Autodesk Inventor part; units mm, degrees
(part 2 of 3)
ref_plane "to_Bolt_1_26_ZX" through (-239.759, 0, -300) normal (0, 0, -1) x (0, 1, 0)
ref_plane "to_Bolt_1_260_XY" through (-278.3133, 0, 300) normal (0, 1, 0) x (1, 0, 0)
ref_plane "to_Bolt_1_260_YZ" through (-278.3133, 0, 300) normal (1, 0, 0) x (0, 0, -1)
ref_plane "to_Bolt_1_260_ZX" through (-278.3133, 0, 300) normal (0, 0, -1) x (0, 1, 0)
ref_plane "to_Bolt_1_261_XY" through (-275.9036, 0, 300) normal (0, 1, 0) x (1, 0, 0)
ref_plane "to_Bolt_1_261_YZ" through (-275.9036, 0, 300) normal (1, 0, 0) x (0, 0, -1)
ref_plane "to_Bolt_1_261_ZX" through (-275.9036, 0, 300) normal (0, 0, -1) x (0, 1, 0)
ref_plane "to_Bolt_1_262_XY" through (-273.494, 0, 300) normal (0, 1, 0) x (1, 0, 0)
ref_plane "to_Bolt_1_262_YZ" through (-273.494, 0, 300) normal (1, 0, 0) x (0, 0, -1)
ref_plane "to_Bolt_1_262_ZX" through (-273.494, 0, 300) normal (0, 0, -1) x (0, 1, 0)
ref_plane "to_Bolt_1_263_XY" through (-271.0843, 0, 300) normal (0, 1, 0) x (1, 0, 0)
ref_plane "to_Bolt_1_263_YZ" through (-271.0843, 0, 300) normal (1, 0, 0) x (0, 0, -1)
ref_plane "to_Bolt_1_263_ZX" through (-271.0843, 0, 300) normal (0, 0, -1) x (0, 1, 0)
ref_plane "to_Bolt_1_264_XY" through (-268.6747, 0, 300) normal (0, 1, 0) x (1, 0, 0)
ref_plane "to_Bolt_1_264_YZ" through (-268.6747, 0, 300) normal (1, 0, 0) x (0, 0, -1)
ref_plane "to_Bolt_1_264_ZX" through (-268.6747, 0, 300) normal (0, 0, -1) x (0, 1, 0)
ref_plane "to_Bolt_1_265_XY" through (-266.2651, 0, 300) normal (0, 1, 0) x (1, 0, 0)
ref_plane "to_Bolt_1_265_YZ" through (-266.2651, 0, 300) normal (1, 0, 0) x (0, 0, -1)
ref_plane "to_Bolt_1_265_ZX" through (-266.2651, 0, 300) normal (0, 0, -1) x (0, 1, 0)
ref_plane "to_Bolt_1_266_XY" through (-263.8554, 0, 300) normal (0, 1, 0) x (1, 0, 0)
ref_plane "to_Bolt_1_266_YZ" through (-263.8554, 0, 300) normal (1, 0, 0) x (0, 0, -1)
ref_plane "to_Bolt_1_266_ZX" through (-263.8554, 0, 300) normal (0, 0, -1) x (0, 1, 0)
ref_plane "to_Bolt_1_267_XY" through (-261.4458, 0, 300) normal (0, 1, 0) x (1, 0, 0)
ref_plane "to_Bolt_1_267_YZ" through (-261.4458, 0, 300) normal (1, 0, 0) x (0, 0, -1)
ref_plane "to_Bolt_1_267_ZX" through (-261.4458, 0, 300) normal (0, 0, -1) x (0, 1, 0)
ref_plane "to_Bolt_1_268_XY" through (-259.0361, 0, 300) normal (0, 1, 0) x (1, 0, 0)
ref_plane "to_Bolt_1_268_YZ" through (-259.0361, 0, 300) normal (1, 0, 0) x (0, 0, -1)
ref_plane "to_Bolt_1_268_ZX" through (-259.0361, 0, 300) normal (0, 0, -1) x (0, 1, 0)
ref_plane "to_Bolt_1_269_XY" through (-256.6265, 0, 300) normal (0, 1, 0) x (1, 0, 0)
ref_plane "to_Bolt_1_269_YZ" through (-256.6265, 0, 300) normal (1, 0, 0) x (0, 0, -1)
ref_plane "to_Bolt_1_269_ZX" through (-256.6265, 0, 300) normal (0, 0, -1) x (0, 1, 0)
ref_plane "to_Bolt_1_27_XY" through (-237.3494, 0, -300) normal (0, 1, 0) x (1, 0, 0)
ref_plane "to_Bolt_1_27_YZ" through (-237.3494, 0, -300) normal (1, 0, 0) x (0, 0, -1)
ref_plane "to_Bolt_1_27_ZX" through (-237.3494, 0, -300) normal (0, 0, -1) x (0, 1, 0)
ref_plane "to_Bolt_1_270_XY" through (-254.2169, 0, 300) normal (0, 1, 0) x (1, 0, 0)
ref_plane "to_Bolt_1_270_YZ" through (-254.2169, 0, 300) normal (1, 0, 0) x (0, 0, -1)
ref_plane "to_Bolt_1_270_ZX" through (-254.2169, 0, 300) normal (0, 0, -1) x (0, 1, 0)
ref_plane "to_Bolt_1_271_XY" through (-251.8072, 0, 300) normal (0, 1, 0) x (1, 0, 0)
ref_plane "to_Bolt_1_271_YZ" through (-251.8072, 0, 300) normal (1, 0, 0) x (0, 0, -1)
ref_plane "to_Bolt_1_271_ZX" through (-251.8072, 0, 300) normal (0, 0, -1) x (0, 1, 0)
ref_plane "to_Bolt_1_272_XY" through (-249.3976, 0, 300) normal (0, 1, 0) x (1, 0, 0)
ref_plane "to_Bolt_1_272_YZ" through (-249.3976, 0, 300) normal (1, 0, 0) x (0, 0, -1)
ref_plane "to_Bolt_1_272_ZX" through (-249.3976, 0, 300) normal (0, 0, -1) x (0, 1, 0)
ref_plane "to_Bolt_1_273_XY" through (-246.988, 0, 300) normal (0, 1, 0) x (1, 0, 0)
ref_plane "to_Bolt_1_273_YZ" through (-246.988, 0, 300) normal (1, 0, 0) x (0, 0, -1)
ref_plane "to_Bolt_1_273_ZX" through (-246.988, 0, 300) normal (0, 0, -1) x (0, 1, 0)
ref_plane "to_Bolt_1_274_XY" through (-244.5783, 0, 300) normal (0, 1, 0) x (1, 0, 0)
ref_plane "to_Bolt_1_274_YZ" through (-244.5783, 0, 300) normal (1, 0, 0) x (0, 0, -1)
ref_plane "to_Bolt_1_274_ZX" through (-244.5783, 0, 300) normal (0, 0, -1) x (0, 1, 0)
ref_plane "to_Bolt_1_275_XY" through (-242.1687, 0, 300) normal (0, 1, 0) x (1, 0, 0)
ref_plane "to_Bolt_1_275_YZ" through (-242.1687, 0, 300) normal (1, 0, 0) x (0, 0, -1)
ref_plane "to_Bolt_1_275_ZX" through (-242.1687, 0, 300) normal (0, 0, -1) x (0, 1, 0)
ref_plane "to_Bolt_1_276_XY" through (-239.759, 0, 300) normal (0, 1, 0) x (1, 0, 0)
ref_plane "to_Bolt_1_276_YZ" through (-239.759, 0, 300) normal (1, 0, 0) x (0, 0, -1)
ref_plane "to_Bolt_1_276_ZX" through (-239.759, 0, 300) normal (0, 0, -1) x (0, 1, 0)
ref_plane "to_Bolt_1_277_XY" through (-237.3494, 0, 300) normal (0, 1, 0) x (1, 0, 0)
ref_plane "to_Bolt_1_277_YZ" through (-237.3494, 0, 300) normal (1, 0, 0) x (0, 0, -1)
ref_plane "to_Bolt_1_277_ZX" through (-237.3494, 0, 300) normal (0, 0, -1) x (0, 1, 0)
ref_plane "to_Bolt_1_278_XY" through (-234.9398, 0, 300) normal (0, 1, 0) x (1, 0, 0)
ref_plane "to_Bolt_1_278_YZ" through (-234.9398, 0, 300) normal (1, 0, 0) x (0, 0, -1)
ref_plane "to_Bolt_1_278_ZX" through (-234.9398, 0, 300) normal (0, 0, -1) x (0, 1, 0)
ref_plane "to_Bolt_1_279_XY" through (-232.5301, 0, 300) normal (0, 1, 0) x (1, 0, 0)
ref_plane "to_Bolt_1_279_YZ" through (-232.5301, 0, 300) normal (1, 0, 0) x (0, 0, -1)
ref_plane "to_Bolt_1_279_ZX" through (-232.5301, 0, 300) normal (0, 0, -1) x (0, 1, 0)
ref_plane "to_Bolt_1_28_XY" through (-234.9398, 0, -300) normal (0, 1, 0) x (1, 0, 0)
ref_plane "to_Bolt_1_28_YZ" through (-234.9398, 0, -300) normal (1, 0, 0) x (0, 0, -1)
ref_plane "to_Bolt_1_28_ZX" through (-234.9398, 0, -300) normal (0, 0, -1) x (0, 1, 0)
ref_plane "to_Bolt_1_280_XY" through (-230.1205, 0, 300) normal (0, 1, 0) x (1, 0, 0)
ref_plane "to_Bolt_1_280_YZ" through (-230.1205, 0, 300) normal (1, 0, 0) x (0, 0, -1)
ref_plane "to_Bolt_1_280_ZX" through (-230.1205, 0, 300) normal (0, 0, -1) x (0, 1, 0)
ref_plane "to_Bolt_1_281_XY" through (-227.7108, 0, 300) normal (0, 1, 0) x (1, 0, 0)
ref_plane "to_Bolt_1_281_YZ" through (-227.7108, 0, 300) normal (1, 0, 0) x (0, 0, -1)
ref_plane "to_Bolt_1_281_ZX" through (-227.7108, 0, 300) normal (0, 0, -1) x (0, 1, 0)
ref_plane "to_Bolt_1_282_XY" through (-225.3012, 0, 300) normal (0, 1, 0) x (1, 0, 0)
ref_plane "to_Bolt_1_282_YZ" through (-225.3012, 0, 300) normal (1, 0, 0) x (0, 0, -1)
ref_plane "to_Bolt_1_282_ZX" through (-225.3012, 0, 300) normal (0, 0, -1) x (0, 1, 0)
ref_plane "to_Bolt_1_283_XY" through (-222.8916, 0, 300) normal (0, 1, 0) x (1, 0, 0)
ref_plane "to_Bolt_1_283_YZ" through (-222.8916, 0, 300) normal (1, 0, 0) x (0, 0, -1)
ref_plane "to_Bolt_1_283_ZX" through (-222.8916, 0, 300) normal (0, 0, -1) x (0, 1, 0)
ref_plane "to_Bolt_1_284_XY" through (-220.4819, 0, 300) normal (0, 1, 0) x (1, 0, 0)
ref_plane "to_Bolt_1_284_YZ" through (-220.4819, 0, 300) normal (1, 0, 0) x (0, 0, -1)
ref_plane "to_Bolt_1_284_ZX" through (-220.4819, 0, 300) normal (0, 0, -1) x (0, 1, 0)
ref_plane "to_Bolt_1_285_XY" through (-218.0723, 0, 300) normal (0, 1, 0) x (1, 0, 0)
ref_plane "to_Bolt_1_285_YZ" through (-218.0723, 0, 300) normal (1, 0, 0) x (0, 0, -1)
ref_plane "to_Bolt_1_285_ZX" through (-218.0723, 0, 300) normal (0, 0, -1) x (0, 1, 0)
ref_plane "to_Bolt_1_286_XY" through (-215.6627, 0, 300) normal (0, 1, 0) x (1, 0, 0)
ref_plane "to_Bolt_1_286_YZ" through (-215.6627, 0, 300) normal (1, 0, 0) x (0, 0, -1)
ref_plane "to_Bolt_1_286_ZX" through (-215.6627, 0, 300) normal (0, 0, -1) x (0, 1, 0)
ref_plane "to_Bolt_1_287_XY" through (-213.253, 0, 300) normal (0, 1, 0) x (1, 0, 0)
ref_plane "to_Bolt_1_287_YZ" through (-213.253, 0, 300) normal (1, 0, 0) x (0, 0, -1)
ref_plane "to_Bolt_1_287_ZX" through (-213.253, 0, 300) normal (0, 0, -1) x (0, 1, 0)
ref_plane "to_Bolt_1_288_XY" through (-210.8434, 0, 300) normal (0, 1, 0) x (1, 0, 0)
ref_plane "to_Bolt_1_288_YZ" through (-210.8434, 0, 300) normal (1, 0, 0) x (0, 0, -1)
ref_plane "to_Bolt_1_288_ZX" through (-210.8434, 0, 300) normal (0, 0, -1) x (0, 1, 0)
ref_plane "to_Bolt_1_289_XY" through (-208.4337, 0, 300) normal (0, 1, 0) x (1, 0, 0)
ref_plane "to_Bolt_1_289_YZ" through (-208.4337, 0, 300) normal (1, 0, 0) x (0, 0, -1)
ref_plane "to_Bolt_1_289_ZX" through (-208.4337, 0, 300) normal (0, 0, -1) x (0, 1, 0)
ref_plane "to_Bolt_1_29_XY" through (-232.5301, 0, -300) normal (0, 1, 0) x (1, 0, 0)
ref_plane "to_Bolt_1_29_YZ" through (-232.5301, 0, -300) normal (1, 0, 0) x (0, 0, -1)
ref_plane "to_Bolt_1_29_ZX" through (-232.5301, 0, -300) normal (0, 0, -1) x (0, 1, 0)
ref_plane "to_Bolt_1_290_XY" through (-206.0241, 0, 300) normal (0, 1, 0) x (1, 0, 0)
ref_plane "to_Bolt_1_290_YZ" through (-206.0241, 0, 300) normal (1, 0, 0) x (0, 0, -1)
ref_plane "to_Bolt_1_290_ZX" through (-206.0241, 0, 300) normal (0, 0, -1) x (0, 1, 0)
ref_plane "to_Bolt_1_291_XY" through (-203.6145, 0, 300) normal (0, 1, 0) x (1, 0, 0)
ref_plane "to_Bolt_1_291_YZ" through (-203.6145, 0, 300) normal (1, 0, 0) x (0, 0, -1)
ref_plane "to_Bolt_1_291_ZX" through (-203.6145, 0, 300) normal (0, 0, -1) x (0, 1, 0)
ref_plane "to_Bolt_1_292_XY" through (-201.2048, 0, 300) normal (0, 1, 0) x (1, 0, 0)
ref_plane "to_Bolt_1_292_YZ" through (-201.2048, 0, 300) normal (1, 0, 0) x (0, 0, -1)
ref_plane "to_Bolt_1_292_ZX" through (-201.2048, 0, 300) normal (0, 0, -1) x (0, 1, 0)
ref_plane "to_Bolt_1_293_XY" through (-198.7952, 0, 300) normal (0, 1, 0) x (1, 0, 0)
ref_plane "to_Bolt_1_293_YZ" through (-198.7952, 0, 300) normal (1, 0, 0) x (0, 0, -1)
ref_plane "to_Bolt_1_293_ZX" through (-198.7952, 0, 300) normal (0, 0, -1) x (0, 1, 0)
ref_plane "to_Bolt_1_294_XY" through (-196.3855, 0, 300) normal (0, 1, 0) x (1, 0, 0)
ref_plane "to_Bolt_1_294_YZ" through (-196.3855, 0, 300) normal (1, 0, 0) x (0, 0, -1)
ref_plane "to_Bolt_1_294_ZX" through (-196.3855, 0, 300) normal (0, 0, -1) x (0, 1, 0)
ref_plane "to_Bolt_1_295_XY" through (-193.9759, 0, 300) normal (0, 1, 0) x (1, 0, 0)
ref_plane "to_Bolt_1_295_YZ" through (-193.9759, 0, 300) normal (1, 0, 0) x (0, 0, -1)
ref_plane "to_Bolt_1_295_ZX" through (-193.9759, 0, 300) normal (0, 0, -1) x (0, 1, 0)
ref_plane "to_Bolt_1_296_XY" through (-191.5663, 0, 300) normal (0, 1, 0) x (1, 0, 0)
ref_plane "to_Bolt_1_296_YZ" through (-191.5663, 0, 300) normal (1, 0, 0) x (0, 0, -1)
ref_plane "to_Bolt_1_296_ZX" through (-191.5663, 0, 300) normal (0, 0, -1) x (0, 1, 0)
ref_plane "to_Bolt_1_297_XY" through (-189.1566, 0, 300) normal (0, 1, 0) x (1, 0, 0)
ref_plane "to_Bolt_1_297_YZ" through (-189.1566, 0, 300) normal (1, 0, 0) x (0, 0, -1)
ref_plane "to_Bolt_1_297_ZX" through (-189.1566, 0, 300) normal (0, 0, -1) x (0, 1, 0)
ref_plane "to_Bolt_1_298_XY" through (-186.747, 0, 300) normal (0, 1, 0) x (1, 0, 0)
ref_plane "to_Bolt_1_298_YZ" through (-186.747, 0, 300) normal (1, 0, 0) x (0, 0, -1)
ref_plane "to_Bolt_1_298_ZX" through (-186.747, 0, 300) normal (0, 0, -1) x (0, 1, 0)
ref_plane "to_Bolt_1_299_XY" through (-184.3373, 0, 300) normal (0, 1, 0) x (1, 0, 0)
ref_plane "to_Bolt_1_299_YZ" through (-184.3373, 0, 300) normal (1, 0, 0) x (0, 0, -1)
ref_plane "to_Bolt_1_299_ZX" through (-184.3373, 0, 300) normal (0, 0, -1) x (0, 1, 0)
ref_plane "to_Bolt_1_3_XY" through (-295.1807, 0, -300) normal (0, 1, 0) x (1, 0, 0)
ref_plane "to_Bolt_1_3_YZ" through (-295.1807, 0, -300) normal (1, 0, 0) x (0, 0, -1)
ref_plane "to_Bolt_1_3_ZX" through (-295.1807, 0, -300) normal (0, 0, -1) x (0, 1, 0)
ref_plane "to_Bolt_1_30_XY" through (-230.1205, 0, -300) normal (0, 1, 0) x (1, 0, 0)
ref_plane "to_Bolt_1_30_YZ" through (-230.1205, 0, -300) normal (1, 0, 0) x (0, 0, -1)
ref_plane "to_Bolt_1_30_ZX" through (-230.1205, 0, -300) normal (0, 0, -1) x (0, 1, 0)
ref_plane "to_Bolt_1_300_XY" through (-181.9277, 0, 300) normal (0, 1, 0) x (1, 0, 0)
ref_plane "to_Bolt_1_300_YZ" through (-181.9277, 0, 300) normal (1, 0, 0) x (0, 0, -1)
ref_plane "to_Bolt_1_300_ZX" through (-181.9277, 0, 300) normal (0, 0, -1) x (0, 1, 0)
ref_plane "to_Bolt_1_301_XY" through (-179.5181, 0, 300) normal (0, 1, 0) x (1, 0, 0)
ref_plane "to_Bolt_1_301_YZ" through (-179.5181, 0, 300) normal (1, 0, 0) x (0, 0, -1)
ref_plane "to_Bolt_1_301_ZX" through (-179.5181, 0, 300) normal (0, 0, -1) x (0, 1, 0)
ref_plane "to_Bolt_1_302_XY" through (-177.1084, 0, 300) normal (0, 1, 0) x (1, 0, 0)
ref_plane "to_Bolt_1_302_YZ" through (-177.1084, 0, 300) normal (1, 0, 0) x (0, 0, -1)
ref_plane "to_Bolt_1_302_ZX" through (-177.1084, 0, 300) normal (0, 0, -1) x (0, 1, 0)
ref_plane "to_Bolt_1_303_XY" through (-174.6988, 0, 300) normal (0, 1, 0) x (1, 0, 0)
ref_plane "to_Bolt_1_303_YZ" through (-174.6988, 0, 300) normal (1, 0, 0) x (0, 0, -1)
ref_plane "to_Bolt_1_303_ZX" through (-174.6988, 0, 300) normal (0, 0, -1) x (0, 1, 0)
ref_plane "to_Bolt_1_304_XY" through (-172.2892, 0, 300) normal (0, 1, 0) x (1, 0, 0)
ref_plane "to_Bolt_1_304_YZ" through (-172.2892, 0, 300) normal (1, 0, 0) x (0, 0, -1)
ref_plane "to_Bolt_1_304_ZX" through (-172.2892, 0, 300) normal (0, 0, -1) x (0, 1, 0)
ref_plane "to_Bolt_1_305_XY" through (-169.8795, 0, 300) normal (0, 1, 0) x (1, 0, 0)
ref_plane "to_Bolt_1_305_YZ" through (-169.8795, 0, 300) normal (1, 0, 0) x (0, 0, -1)
ref_plane "to_Bolt_1_305_ZX" through (-169.8795, 0, 300) normal (0, 0, -1) x (0, 1, 0)
ref_plane "to_Bolt_1_306_XY" through (-167.4699, 0, 300) normal (0, 1, 0) x (1, 0, 0)
ref_plane "to_Bolt_1_306_YZ" through (-167.4699, 0, 300) normal (1, 0, 0) x (0, 0, -1)
ref_plane "to_Bolt_1_306_ZX" through (-167.4699, 0, 300) normal (0, 0, -1) x (0, 1, 0)
ref_plane "to_Bolt_1_307_XY" through (-165.0602, 0, 300) normal (0, 1, 0) x (1, 0, 0)
ref_plane "to_Bolt_1_307_YZ" through (-165.0602, 0, 300) normal (1, 0, 0) x (0, 0, -1)
ref_plane "to_Bolt_1_307_ZX" through (-165.0602, 0, 300) normal (0, 0, -1) x (0, 1, 0)
ref_plane "to_Bolt_1_308_XY" through (-162.6506, 0, 300) normal (0, 1, 0) x (1, 0, 0)
ref_plane "to_Bolt_1_308_YZ" through (-162.6506, 0, 300) normal (1, 0, 0) x (0, 0, -1)
ref_plane "to_Bolt_1_308_ZX" through (-162.6506, 0, 300) normal (0, 0, -1) x (0, 1, 0)
ref_plane "to_Bolt_1_309_XY" through (-160.241, 0, 300) normal (0, 1, 0) x (1, 0, 0)
ref_plane "to_Bolt_1_309_YZ" through (-160.241, 0, 300) normal (1, 0, 0) x (0, 0, -1)
ref_plane "to_Bolt_1_309_ZX" through (-160.241, 0, 300) normal (0, 0, -1) x (0, 1, 0)
ref_plane "to_Bolt_1_31_XY" through (-227.7108, 0, -300) normal (0, 1, 0) x (1, 0, 0)
ref_plane "to_Bolt_1_31_YZ" through (-227.7108, 0, -300) normal (1, 0, 0) x (0, 0, -1)
ref_plane "to_Bolt_1_31_ZX" through (-227.7108, 0, -300) normal (0, 0, -1) x (0, 1, 0)
ref_plane "to_Bolt_1_310_XY" through (-157.8313, 0, 300) normal (0, 1, 0) x (1, 0, 0)
ref_plane "to_Bolt_1_310_YZ" through (-157.8313, 0, 300) normal (1, 0, 0) x (0, 0, -1)
ref_plane "to_Bolt_1_310_ZX" through (-157.8313, 0, 300) normal (0, 0, -1) x (0, 1, 0)
ref_plane "to_Bolt_1_311_XY" through (-155.4217, 0, 300) normal (0, 1, 0) x (1, 0, 0)
ref_plane "to_Bolt_1_311_YZ" through (-155.4217, 0, 300) normal (1, 0, 0) x (0, 0, -1)
ref_plane "to_Bolt_1_311_ZX" through (-155.4217, 0, 300) normal (0, 0, -1) x (0, 1, 0)
ref_plane "to_Bolt_1_312_XY" through (-153.012, 0, 300) normal (0, 1, 0) x (1, 0, 0)
ref_plane "to_Bolt_1_312_YZ" through (-153.012, 0, 300) normal (1, 0, 0) x (0, 0, -1)
ref_plane "to_Bolt_1_312_ZX" through (-153.012, 0, 300) normal (0, 0, -1) x (0, 1, 0)
ref_plane "to_Bolt_1_313_XY" through (-150.6024, 0, 300) normal (0, 1, 0) x (1, 0, 0)
ref_plane "to_Bolt_1_313_YZ" through (-150.6024, 0, 300) normal (1, 0, 0) x (0, 0, -1)
ref_plane "to_Bolt_1_313_ZX" through (-150.6024, 0, 300) normal (0, 0, -1) x (0, 1, 0)
ref_plane "to_Bolt_1_314_XY" through (-148.1928, 0, 300) normal (0, 1, 0) x (1, 0, 0)
ref_plane "to_Bolt_1_314_YZ" through (-148.1928, 0, 300) normal (1, 0, 0) x (0, 0, -1)
ref_plane "to_Bolt_1_314_ZX" through (-148.1928, 0, 300) normal (0, 0, -1) x (0, 1, 0)
ref_plane "to_Bolt_1_315_XY" through (-145.7831, 0, 300) normal (0, 1, 0) x (1, 0, 0)
ref_plane "to_Bolt_1_315_YZ" through (-145.7831, 0, 300) normal (1, 0, 0) x (0, 0, -1)
ref_plane "to_Bolt_1_315_ZX" through (-145.7831, 0, 300) normal (0, 0, -1) x (0, 1, 0)
ref_plane "to_Bolt_1_316_XY" through (-143.3735, 0, 300) normal (0, 1, 0) x (1, 0, 0)
ref_plane "to_Bolt_1_316_YZ" through (-143.3735, 0, 300) normal (1, 0, 0) x (0, 0, -1)
ref_plane "to_Bolt_1_316_ZX" through (-143.3735, 0, 300) normal (0, 0, -1) x (0, 1, 0)
ref_plane "to_Bolt_1_317_XY" through (-140.9639, 0, 300) normal (0, 1, 0) x (1, 0, 0)
ref_plane "to_Bolt_1_317_YZ" through (-140.9639, 0, 300) normal (1, 0, 0) x (0, 0, -1)
ref_plane "to_Bolt_1_317_ZX" through (-140.9639, 0, 300) normal (0, 0, -1) x (0, 1, 0)
ref_plane "to_Bolt_1_318_XY" through (-138.5542, 0, 300) normal (0, 1, 0) x (1, 0, 0)
ref_plane "to_Bolt_1_318_YZ" through (-138.5542, 0, 300) normal (1, 0, 0) x (0, 0, -1)
ref_plane "to_Bolt_1_318_ZX" through (-138.5542, 0, 300) normal (0, 0, -1) x (0, 1, 0)
ref_plane "to_Bolt_1_319_XY" through (-136.1446, 0, 300) normal (0, 1, 0) x (1, 0, 0)
ref_plane "to_Bolt_1_319_YZ" through (-136.1446, 0, 300) normal (1, 0, 0) x (0, 0, -1)
ref_plane "to_Bolt_1_319_ZX" through (-136.1446, 0, 300) normal (0, 0, -1) x (0, 1, 0)
ref_plane "to_Bolt_1_32_XY" through (-225.3012, 0, -300) normal (0, 1, 0) x (1, 0, 0)
ref_plane "to_Bolt_1_32_YZ" through (-225.3012, 0, -300) normal (1, 0, 0) x (0, 0, -1)
ref_plane "to_Bolt_1_32_ZX" through (-225.3012, 0, -300) normal (0, 0, -1) x (0, 1, 0)
ref_plane "to_Bolt_1_320_XY" through (-133.7349, 0, 300) normal (0, 1, 0) x (1, 0, 0)
ref_plane "to_Bolt_1_320_YZ" through (-133.7349, 0, 300) normal (1, 0, 0) x (0, 0, -1)
ref_plane "to_Bolt_1_320_ZX" through (-133.7349, 0, 300) normal (0, 0, -1) x (0, 1, 0)
ref_plane "to_Bolt_1_321_XY" through (-131.3253, 0, 300) normal (0, 1, 0) x (1, 0, 0)
ref_plane "to_Bolt_1_321_YZ" through (-131.3253, 0, 300) normal (1, 0, 0) x (0, 0, -1)
ref_plane "to_Bolt_1_321_ZX" through (-131.3253, 0, 300) normal (0, 0, -1) x (0, 1, 0)
ref_plane "to_Bolt_1_322_XY" through (-128.9157, 0, 300) normal (0, 1, 0) x (1, 0, 0)
ref_plane "to_Bolt_1_322_YZ" through (-128.9157, 0, 300) normal (1, 0, 0) x (0, 0, -1)
ref_plane "to_Bolt_1_322_ZX" through (-128.9157, 0, 300) normal (0, 0, -1) x (0, 1, 0)
ref_plane "to_Bolt_1_323_XY" through (-126.506, 0, 300) normal (0, 1, 0) x (1, 0, 0)
ref_plane "to_Bolt_1_323_YZ" through (-126.506, 0, 300) normal (1, 0, 0) x (0, 0, -1)
ref_plane "to_Bolt_1_323_ZX" through (-126.506, 0, 300) normal (0, 0, -1) x (0, 1, 0)
ref_plane "to_Bolt_1_324_XY" through (-124.0964, 0, 300) normal (0, 1, 0) x (1, 0, 0)
ref_plane "to_Bolt_1_324_YZ" through (-124.0964, 0, 300) normal (1, 0, 0) x (0, 0, -1)
ref_plane "to_Bolt_1_324_ZX" through (-124.0964, 0, 300) normal (0, 0, -1) x (0, 1, 0)
ref_plane "to_Bolt_1_325_XY" through (-121.6867, 0, 300) normal (0, 1, 0) x (1, 0, 0)
ref_plane "to_Bolt_1_325_YZ" through (-121.6867, 0, 300) normal (1, 0, 0) x (0, 0, -1)
ref_plane "to_Bolt_1_325_ZX" through (-121.6867, 0, 300) normal (0, 0, -1) x (0, 1, 0)
ref_plane "to_Bolt_1_326_XY" through (-119.2771, 0, 300) normal (0, 1, 0) x (1, 0, 0)
ref_plane "to_Bolt_1_326_YZ" through (-119.2771, 0, 300) normal (1, 0, 0) x (0, 0, -1)
ref_plane "to_Bolt_1_326_ZX" through (-119.2771, 0, 300) normal (0, 0, -1) x (0, 1, 0)
ref_plane "to_Bolt_1_327_XY" through (-116.8675, 0, 300) normal (0, 1, 0) x (1, 0, 0)
ref_plane "to_Bolt_1_327_YZ" through (-116.8675, 0, 300) normal (1, 0, 0) x (0, 0, -1)
ref_plane "to_Bolt_1_327_ZX" through (-116.8675, 0, 300) normal (0, 0, -1) x (0, 1, 0)
ref_plane "to_Bolt_1_328_XY" through (-114.4578, 0, 300) normal (0, 1, 0) x (1, 0, 0)
ref_plane "to_Bolt_1_328_YZ" through (-114.4578, 0, 300) normal (1, 0, 0) x (0, 0, -1)
ref_plane "to_Bolt_1_328_ZX" through (-114.4578, 0, 300) normal (0, 0, -1) x (0, 1, 0)
ref_plane "to_Bolt_1_329_XY" through (-112.0482, 0, 300) normal (0, 1, 0) x (1, 0, 0)
ref_plane "to_Bolt_1_329_YZ" through (-112.0482, 0, 300) normal (1, 0, 0) x (0, 0, -1)
ref_plane "to_Bolt_1_329_ZX" through (-112.0482, 0, 300) normal (0, 0, -1) x (0, 1, 0)
ref_plane "to_Bolt_1_33_XY" through (-222.8916, 0, -300) normal (0, 1, 0) x (1, 0, 0)
ref_plane "to_Bolt_1_33_YZ" through (-222.8916, 0, -300) normal (1, 0, 0) x (0, 0, -1)
ref_plane "to_Bolt_1_33_ZX" through (-222.8916, 0, -300) normal (0, 0, -1) x (0, 1, 0)
ref_plane "to_Bolt_1_330_XY" through (-109.6386, 0, 300) normal (0, 1, 0) x (1, 0, 0)
ref_plane "to_Bolt_1_330_YZ" through (-109.6386, 0, 300) normal (1, 0, 0) x (0, 0, -1)
ref_plane "to_Bolt_1_330_ZX" through (-109.6386, 0, 300) normal (0, 0, -1) x (0, 1, 0)
ref_plane "to_Bolt_1_331_XY" through (-107.2289, 0, 300) normal (0, 1, 0) x (1, 0, 0)
ref_plane "to_Bolt_1_331_YZ" through (-107.2289, 0, 300) normal (1, 0, 0) x (0, 0, -1)
ref_plane "to_Bolt_1_331_ZX" through (-107.2289, 0, 300) normal (0, 0, -1) x (0, 1, 0)
ref_plane "to_Bolt_1_332_XY" through (-104.8193, 0, 300) normal (0, 1, 0) x (1, 0, 0)
ref_plane "to_Bolt_1_332_YZ" through (-104.8193, 0, 300) normal (1, 0, 0) x (0, 0, -1)
ref_plane "to_Bolt_1_332_ZX" through (-104.8193, 0, 300) normal (0, 0, -1) x (0, 1, 0)
ref_plane "to_Bolt_1_333_XY" through (-102.4096, 0, 300) normal (0, 1, 0) x (1, 0, 0)
ref_plane "to_Bolt_1_333_YZ" through (-102.4096, 0, 300) normal (1, 0, 0) x (0, 0, -1)
ref_plane "to_Bolt_1_333_ZX" through (-102.4096, 0, 300) normal (0, 0, -1) x (0, 1, 0)
ref_plane "to_Bolt_1_334_XY" through (-100, 0, 300) normal (0, 1, 0) x (1, 0, 0)
ref_plane "to_Bolt_1_334_YZ" through (-100, 0, 300) normal (1, 0, 0) x (0, 0, -1)
ref_plane "to_Bolt_1_334_ZX" through (-100, 0, 300) normal (0, 0, -1) x (0, 1, 0)
ref_plane "to_Bolt_1_335_XY" through (-97.5904, 0, 300) normal (0, 1, 0) x (1, 0, 0)
ref_plane "to_Bolt_1_335_YZ" through (-97.5904, 0, 300) normal (1, 0, 0) x (0, 0, -1)
ref_plane "to_Bolt_1_335_ZX" through (-97.5904, 0, 300) normal (0, 0, -1) x (0, 1, 0)
ref_plane "to_Bolt_1_336_XY" through (-95.1807, 0, 300) normal (0, 1, 0) x (1, 0, 0)
ref_plane "to_Bolt_1_336_YZ" through (-95.1807, 0, 300) normal (1, 0, 0) x (0, 0, -1)
ref_plane "to_Bolt_1_336_ZX" through (-95.1807, 0, 300) normal (0, 0, -1) x (0, 1, 0)
ref_plane "to_Bolt_1_337_XY" through (-92.7711, 0, 300) normal (0, 1, 0) x (1, 0, 0)
ref_plane "to_Bolt_1_337_YZ" through (-92.7711, 0, 300) normal (1, 0, 0) x (0, 0, -1)
ref_plane "to_Bolt_1_337_ZX" through (-92.7711, 0, 300) normal (0, 0, -1) x (0, 1, 0)
ref_plane "to_Bolt_1_338_XY" through (-90.3614, 0, 300) normal (0, 1, 0) x (1, 0, 0)
ref_plane "to_Bolt_1_338_YZ" through (-90.3614, 0, 300) normal (1, 0, 0) x (0, 0, -1)
ref_plane "to_Bolt_1_338_ZX" through (-90.3614, 0, 300) normal (0, 0, -1) x (0, 1, 0)
ref_plane "to_Bolt_1_339_XY" through (-87.9518, 0, 300) normal (0, 1, 0) x (1, 0, 0)
ref_plane "to_Bolt_1_339_YZ" through (-87.9518, 0, 300) normal (1, 0, 0) x (0, 0, -1)
ref_plane "to_Bolt_1_339_ZX" through (-87.9518, 0, 300) normal (0, 0, -1) x (0, 1, 0)
ref_plane "to_Bolt_1_34_XY" through (-220.4819, 0, -300) normal (0, 1, 0) x (1, 0, 0)
ref_plane "to_Bolt_1_34_YZ" through (-220.4819, 0, -300) normal (1, 0, 0) x (0, 0, -1)
ref_plane "to_Bolt_1_34_ZX" through (-220.4819, 0, -300) normal (0, 0, -1) x (0, 1, 0)
ref_plane "to_Bolt_1_340_XY" through (-85.5422, 0, 300) normal (0, 1, 0) x (1, 0, 0)
ref_plane "to_Bolt_1_340_YZ" through (-85.5422, 0, 300) normal (1, 0, 0) x (0, 0, -1)
ref_plane "to_Bolt_1_340_ZX" through (-85.5422, 0, 300) normal (0, 0, -1) x (0, 1, 0)
ref_plane "to_Bolt_1_341_XY" through (-83.1325, 0, 300) normal (0, 1, 0) x (1, 0, 0)
ref_plane "to_Bolt_1_341_YZ" through (-83.1325, 0, 300) normal (1, 0, 0) x (0, 0, -1)
ref_plane "to_Bolt_1_341_ZX" through (-83.1325, 0, 300) normal (0, 0, -1) x (0, 1, 0)
ref_plane "to_Bolt_1_342_XY" through (-80.7229, 0, 300) normal (0, 1, 0) x (1, 0, 0)
ref_plane "to_Bolt_1_342_YZ" through (-80.7229, 0, 300) normal (1, 0, 0) x (0, 0, -1)
ref_plane "to_Bolt_1_342_ZX" through (-80.7229, 0, 300) normal (0, 0, -1) x (0, 1, 0)
ref_plane "to_Bolt_1_343_XY" through (-78.3133, 0, 300) normal (0, 1, 0) x (1, 0, 0)
ref_plane "to_Bolt_1_343_YZ" through (-78.3133, 0, 300) normal (1, 0, 0) x (0, 0, -1)
ref_plane "to_Bolt_1_343_ZX" through (-78.3133, 0, 300) normal (0, 0, -1) x (0, 1, 0)
ref_plane "to_Bolt_1_344_XY" through (-75.9036, 0, 300) normal (0, 1, 0) x (1, 0, 0)
ref_plane "to_Bolt_1_344_YZ" through (-75.9036, 0, 300) normal (1, 0, 0) x (0, 0, -1)
ref_plane "to_Bolt_1_344_ZX" through (-75.9036, 0, 300) normal (0, 0, -1) x (0, 1, 0)
ref_plane "to_Bolt_1_345_XY" through (-73.494, 0, 300) normal (0, 1, 0) x (1, 0, 0)
ref_plane "to_Bolt_1_345_YZ" through (-73.494, 0, 300) normal (1, 0, 0) x (0, 0, -1)
ref_plane "to_Bolt_1_345_ZX" through (-73.494, 0, 300) normal (0, 0, -1) x (0, 1, 0)
ref_plane "to_Bolt_1_346_XY" through (-71.0843, 0, 300) normal (0, 1, 0) x (1, 0, 0)
ref_plane "to_Bolt_1_346_YZ" through (-71.0843, 0, 300) normal (1, 0, 0) x (0, 0, -1)
ref_plane "to_Bolt_1_346_ZX" through (-71.0843, 0, 300) normal (0, 0, -1) x (0, 1, 0)
ref_plane "to_Bolt_1_347_XY" through (-68.6747, 0, 300) normal (0, 1, 0) x (1, 0, 0)
ref_plane "to_Bolt_1_347_YZ" through (-68.6747, 0, 300) normal (1, 0, 0) x (0, 0, -1)
ref_plane "to_Bolt_1_347_ZX" through (-68.6747, 0, 300) normal (0, 0, -1) x (0, 1, 0)
ref_plane "to_Bolt_1_348_XY" through (-66.2651, 0, 300) normal (0, 1, 0) x (1, 0, 0)
ref_plane "to_Bolt_1_348_YZ" through (-66.2651, 0, 300) normal (1, 0, 0) x (0, 0, -1)
ref_plane "to_Bolt_1_348_ZX" through (-66.2651, 0, 300) normal (0, 0, -1) x (0, 1, 0)
ref_plane "to_Bolt_1_349_XY" through (-63.8554, 0, 300) normal (0, 1, 0) x (1, 0, 0)
ref_plane "to_Bolt_1_349_YZ" through (-63.8554, 0, 300) normal (1, 0, 0) x (0, 0, -1)
ref_plane "to_Bolt_1_349_ZX" through (-63.8554, 0, 300) normal (0, 0, -1) x (0, 1, 0)
ref_plane "to_Bolt_1_35_XY" through (-218.0723, 0, -300) normal (0, 1, 0) x (1, 0, 0)
ref_plane "to_Bolt_1_35_YZ" through (-218.0723, 0, -300) normal (1, 0, 0) x (0, 0, -1)
ref_plane "to_Bolt_1_35_ZX" through (-218.0723, 0, -300) normal (0, 0, -1) x (0, 1, 0)
ref_plane "to_Bolt_1_350_XY" through (-61.4458, 0, 300) normal (0, 1, 0) x (1, 0, 0)
ref_plane "to_Bolt_1_350_YZ" through (-61.4458, 0, 300) normal (1, 0, 0) x (0, 0, -1)
ref_plane "to_Bolt_1_350_ZX" through (-61.4458, 0, 300) normal (0, 0, -1) x (0, 1, 0)
ref_plane "to_Bolt_1_351_XY" through (-59.0361, 0, 300) normal (0, 1, 0) x (1, 0, 0)
ref_plane "to_Bolt_1_351_YZ" through (-59.0361, 0, 300) normal (1, 0, 0) x (0, 0, -1)
ref_plane "to_Bolt_1_351_ZX" through (-59.0361, 0, 300) normal (0, 0, -1) x (0, 1, 0)
ref_plane "to_Bolt_1_352_XY" through (-56.6265, 0, 300) normal (0, 1, 0) x (1, 0, 0)
ref_plane "to_Bolt_1_352_YZ" through (-56.6265, 0, 300) normal (1, 0, 0) x (0, 0, -1)
ref_plane "to_Bolt_1_352_ZX" through (-56.6265, 0, 300) normal (0, 0, -1) x (0, 1, 0)
ref_plane "to_Bolt_1_353_XY" through (-54.2169, 0, 300) normal (0, 1, 0) x (1, 0, 0)
ref_plane "to_Bolt_1_353_YZ" through (-54.2169, 0, 300) normal (1, 0, 0) x (0, 0, -1)
ref_plane "to_Bolt_1_353_ZX" through (-54.2169, 0, 300) normal (0, 0, -1) x (0, 1, 0)
ref_plane "to_Bolt_1_354_XY" through (-51.8072, 0, 300) normal (0, 1, 0) x (1, 0, 0)
ref_plane "to_Bolt_1_354_YZ" through (-51.8072, 0, 300) normal (1, 0, 0) x (0, 0, -1)
ref_plane "to_Bolt_1_354_ZX" through (-51.8072, 0, 300) normal (0, 0, -1) x (0, 1, 0)
ref_plane "to_Bolt_1_355_XY" through (-49.3976, 0, 300) normal (0, 1, 0) x (1, 0, 0)
ref_plane "to_Bolt_1_355_YZ" through (-49.3976, 0, 300) normal (1, 0, 0) x (0, 0, -1)
ref_plane "to_Bolt_1_355_ZX" through (-49.3976, 0, 300) normal (0, 0, -1) x (0, 1, 0)
ref_plane "to_Bolt_1_356_XY" through (-46.988, 0, 300) normal (0, 1, 0) x (1, 0, 0)
ref_plane "to_Bolt_1_356_YZ" through (-46.988, 0, 300) normal (1, 0, 0) x (0, 0, -1)
ref_plane "to_Bolt_1_356_ZX" through (-46.988, 0, 300) normal (0, 0, -1) x (0, 1, 0)
ref_plane "to_Bolt_1_357_XY" through (-44.5783, 0, 300) normal (0, 1, 0) x (1, 0, 0)
ref_plane "to_Bolt_1_357_YZ" through (-44.5783, 0, 300) normal (1, 0, 0) x (0, 0, -1)
ref_plane "to_Bolt_1_357_ZX" through (-44.5783, 0, 300) normal (0, 0, -1) x (0, 1, 0)
ref_plane "to_Bolt_1_358_XY" through (-42.1687, 0, 300) normal (0, 1, 0) x (1, 0, 0)
ref_plane "to_Bolt_1_358_YZ" through (-42.1687, 0, 300) normal (1, 0, 0) x (0, 0, -1)
ref_plane "to_Bolt_1_358_ZX" through (-42.1687, 0, 300) normal (0, 0, -1) x (0, 1, 0)
ref_plane "to_Bolt_1_359_XY" through (-39.759, 0, 300) normal (0, 1, 0) x (1, 0, 0)
ref_plane "to_Bolt_1_359_YZ" through (-39.759, 0, 300) normal (1, 0, 0) x (0, 0, -1)
ref_plane "to_Bolt_1_359_ZX" through (-39.759, 0, 300) normal (0, 0, -1) x (0, 1, 0)
ref_plane "to_Bolt_1_36_XY" through (-215.6627, 0, -300) normal (0, 1, 0) x (1, 0, 0)
ref_plane "to_Bolt_1_36_YZ" through (-215.6627, 0, -300) normal (1, 0, 0) x (0, 0, -1)
ref_plane "to_Bolt_1_36_ZX" through (-215.6627, 0, -300) normal (0, 0, -1) x (0, 1, 0)
ref_plane "to_Bolt_1_360_XY" through (-37.3494, 0, 300) normal (0, 1, 0) x (1, 0, 0)
ref_plane "to_Bolt_1_360_YZ" through (-37.3494, 0, 300) normal (1, 0, 0) x (0, 0, -1)
ref_plane "to_Bolt_1_360_ZX" through (-37.3494, 0, 300) normal (0, 0, -1) x (0, 1, 0)
ref_plane "to_Bolt_1_361_XY" through (-34.9398, 0, 300) normal (0, 1, 0) x (1, 0, 0)
ref_plane "to_Bolt_1_361_YZ" through (-34.9398, 0, 300) normal (1, 0, 0) x (0, 0, -1)
ref_plane "to_Bolt_1_361_ZX" through (-34.9398, 0, 300) normal (0, 0, -1) x (0, 1, 0)
ref_plane "to_Bolt_1_362_XY" through (-32.5301, 0, 300) normal (0, 1, 0) x (1, 0, 0)
ref_plane "to_Bolt_1_362_YZ" through (-32.5301, 0, 300) normal (1, 0, 0) x (0, 0, -1)
ref_plane "to_Bolt_1_362_ZX" through (-32.5301, 0, 300) normal (0, 0, -1) x (0, 1, 0)
ref_plane "to_Bolt_1_363_XY" through (-30.1205, 0, 300) normal (0, 1, 0) x (1, 0, 0)
ref_plane "to_Bolt_1_363_YZ" through (-30.1205, 0, 300) normal (1, 0, 0) x (0, 0, -1)
ref_plane "to_Bolt_1_363_ZX" through (-30.1205, 0, 300) normal (0, 0, -1) x (0, 1, 0)
ref_plane "to_Bolt_1_364_XY" through (-27.7108, 0, 300) normal (0, 1, 0) x (1, 0, 0)
ref_plane "to_Bolt_1_364_YZ" through (-27.7108, 0, 300) normal (1, 0, 0) x (0, 0, -1)
ref_plane "to_Bolt_1_364_ZX" through (-27.7108, 0, 300) normal (0, 0, -1) x (0, 1, 0)
ref_plane "to_Bolt_1_365_XY" through (-25.3012, 0, 300) normal (0, 1, 0) x (1, 0, 0)
ref_plane "to_Bolt_1_365_YZ" through (-25.3012, 0, 300) normal (1, 0, 0) x (0, 0, -1)
ref_plane "to_Bolt_1_365_ZX" through (-25.3012, 0, 300) normal (0, 0, -1) x (0, 1, 0)
ref_plane "to_Bolt_1_366_XY" through (-22.8916, 0, 300) normal (0, 1, 0) x (1, 0, 0)
ref_plane "to_Bolt_1_366_YZ" through (-22.8916, 0, 300) normal (1, 0, 0) x (0, 0, -1)
ref_plane "to_Bolt_1_366_ZX" through (-22.8916, 0, 300) normal (0, 0, -1) x (0, 1, 0)
ref_plane "to_Bolt_1_367_XY" through (-20.4819, 0, 300) normal (0, 1, 0) x (1, 0, 0)
ref_plane "to_Bolt_1_367_YZ" through (-20.4819, 0, 300) normal (1, 0, 0) x (0, 0, -1)
ref_plane "to_Bolt_1_367_ZX" through (-20.4819, 0, 300) normal (0, 0, -1) x (0, 1, 0)
ref_plane "to_Bolt_1_368_XY" through (-18.0723, 0, 300) normal (0, 1, 0) x (1, 0, 0)
ref_plane "to_Bolt_1_368_YZ" through (-18.0723, 0, 300) normal (1, 0, 0) x (0, 0, -1)
ref_plane "to_Bolt_1_368_ZX" through (-18.0723, 0, 300) normal (0, 0, -1) x (0, 1, 0)
ref_plane "to_Bolt_1_369_XY" through (-15.6627, 0, 300) normal (0, 1, 0) x (1, 0, 0)
ref_plane "to_Bolt_1_369_YZ" through (-15.6627, 0, 300) normal (1, 0, 0) x (0, 0, -1)
ref_plane "to_Bolt_1_369_ZX" through (-15.6627, 0, 300) normal (0, 0, -1) x (0, 1, 0)
ref_plane "to_Bolt_1_37_XY" through (-213.253, 0, -300) normal (0, 1, 0) x (1, 0, 0)
ref_plane "to_Bolt_1_37_YZ" through (-213.253, 0, -300) normal (1, 0, 0) x (0, 0, -1)
ref_plane "to_Bolt_1_37_ZX" through (-213.253, 0, -300) normal (0, 0, -1) x (0, 1, 0)
ref_plane "to_Bolt_1_370_XY" through (-13.253, 0, 300) normal (0, 1, 0) x (1, 0, 0)
ref_plane "to_Bolt_1_370_YZ" through (-13.253, 0, 300) normal (1, 0, 0) x (0, 0, -1)
ref_plane "to_Bolt_1_370_ZX" through (-13.253, 0, 300) normal (0, 0, -1) x (0, 1, 0)
ref_plane "to_Bolt_1_371_XY" through (-10.8434, 0, 300) normal (0, 1, 0) x (1, 0, 0)
ref_plane "to_Bolt_1_371_YZ" through (-10.8434, 0, 300) normal (1, 0, 0) x (0, 0, -1)
ref_plane "to_Bolt_1_371_ZX" through (-10.8434, 0, 300) normal (0, 0, -1) x (0, 1, 0)
ref_plane "to_Bolt_1_372_XY" through (-8.4337, 0, 300) normal (0, 1, 0) x (1, 0, 0)
ref_plane "to_Bolt_1_372_YZ" through (-8.4337, 0, 300) normal (1, 0, 0) x (0, 0, -1)
ref_plane "to_Bolt_1_372_ZX" through (-8.4337, 0, 300) normal (0, 0, -1) x (0, 1, 0)
ref_plane "to_Bolt_1_373_XY" through (-6.0241, 0, 300) normal (0, 1, 0) x (1, 0, 0)
ref_plane "to_Bolt_1_373_YZ" through (-6.0241, 0, 300) normal (1, 0, 0) x (0, 0, -1)
ref_plane "to_Bolt_1_373_ZX" through (-6.0241, 0, 300) normal (0, 0, -1) x (0, 1, 0)
ref_plane "to_Bolt_1_374_XY" through (-3.6145, 0, 300) normal (0, 1, 0) x (1, 0, 0)
ref_plane "to_Bolt_1_374_YZ" through (-3.6145, 0, 300) normal (1, 0, 0) x (0, 0, -1)
ref_plane "to_Bolt_1_374_ZX" through (-3.6145, 0, 300) normal (0, 0, -1) x (0, 1, 0)
ref_plane "to_Bolt_1_375_XY" through (-1.2048, 0, 300) normal (0, 1, 0) x (1, 0, 0)
ref_plane "to_Bolt_1_375_YZ" through (-1.2048, 0, 300) normal (1, 0, 0) x (0, 0, -1)
ref_plane "to_Bolt_1_375_ZX" through (-1.2048, 0, 300) normal (0, 0, -1) x (0, 1, 0)
ref_plane "to_Bolt_1_376_XY" through (1.2048, 0, 300) normal (0, 1, 0) x (1, 0, 0)
ref_plane "to_Bolt_1_376_YZ" through (1.2048, 0, 300) normal (1, 0, 0) x (0, 0, -1)
ref_plane "to_Bolt_1_376_ZX" through (1.2048, 0, 300) normal (0, 0, -1) x (0, 1, 0)
ref_plane "to_Bolt_1_377_XY" through (3.6145, 0, 300) normal (0, 1, 0) x (1, 0, 0)
ref_plane "to_Bolt_1_377_YZ" through (3.6145, 0, 300) normal (1, 0, 0) x (0, 0, -1)
ref_plane "to_Bolt_1_377_ZX" through (3.6145, 0, 300) normal (0, 0, -1) x (0, 1, 0)
ref_plane "to_Bolt_1_378_XY" through (6.0241, 0, 300) normal (0, 1, 0) x (1, 0, 0)
ref_plane "to_Bolt_1_378_YZ" through (6.0241, 0, 300) normal (1, 0, 0) x (0, 0, -1)
ref_plane "to_Bolt_1_378_ZX" through (6.0241, 0, 300) normal (0, 0, -1) x (0, 1, 0)
ref_plane "to_Bolt_1_379_XY" through (8.4337, 0, 300) normal (0, 1, 0) x (1, 0, 0)
ref_plane "to_Bolt_1_379_YZ" through (8.4337, 0, 300) normal (1, 0, 0) x (0, 0, -1)
ref_plane "to_Bolt_1_379_ZX" through (8.4337, 0, 300) normal (0, 0, -1) x (0, 1, 0)
ref_plane "to_Bolt_1_38_XY" through (-210.8434, 0, -300) normal (0, 1, 0) x (1, 0, 0)
ref_plane "to_Bolt_1_38_YZ" through (-210.8434, 0, -300) normal (1, 0, 0) x (0, 0, -1)
ref_plane "to_Bolt_1_38_ZX" through (-210.8434, 0, -300) normal (0, 0, -1) x (0, 1, 0)
ref_plane "to_Bolt_1_380_XY" through (10.8434, 0, 300) normal (0, 1, 0) x (1, 0, 0)
ref_plane "to_Bolt_1_380_YZ" through (10.8434, 0, 300) normal (1, 0, 0) x (0, 0, -1)
ref_plane "to_Bolt_1_380_ZX" through (10.8434, 0, 300) normal (0, 0, -1) x (0, 1, 0)
ref_plane "to_Bolt_1_381_XY" through (13.253, 0, 300) normal (0, 1, 0) x (1, 0, 0)
ref_plane "to_Bolt_1_381_YZ" through (13.253, 0, 300) normal (1, 0, 0) x (0, 0, -1)
ref_plane "to_Bolt_1_381_ZX" through (13.253, 0, 300) normal (0, 0, -1) x (0, 1, 0)
ref_plane "to_Bolt_1_382_XY" through (15.6627, 0, 300) normal (0, 1, 0) x (1, 0, 0)
ref_plane "to_Bolt_1_382_YZ" through (15.6627, 0, 300) normal (1, 0, 0) x (0, 0, -1)
ref_plane "to_Bolt_1_382_ZX" through (15.6627, 0, 300) normal (0, 0, -1) x (0, 1, 0)
ref_plane "to_Bolt_1_383_XY" through (18.0723, 0, 300) normal (0, 1, 0) x (1, 0, 0)
ref_plane "to_Bolt_1_383_YZ" through (18.0723, 0, 300) normal (1, 0, 0) x (0, 0, -1)
ref_plane "to_Bolt_1_383_ZX" through (18.0723, 0, 300) normal (0, 0, -1) x (0, 1, 0)
ref_plane "to_Bolt_1_384_XY" through (20.4819, 0, 300) normal (0, 1, 0) x (1, 0, 0)
ref_plane "to_Bolt_1_384_YZ" through (20.4819, 0, 300) normal (1, 0, 0) x (0, 0, -1)
ref_plane "to_Bolt_1_384_ZX" through (20.4819, 0, 300) normal (0, 0, -1) x (0, 1, 0)
ref_plane "to_Bolt_1_385_XY" through (22.8916, 0, 300) normal (0, 1, 0) x (1, 0, 0)
ref_plane "to_Bolt_1_385_YZ" through (22.8916, 0, 300) normal (1, 0, 0) x (0, 0, -1)
ref_plane "to_Bolt_1_385_ZX" through (22.8916, 0, 300) normal (0, 0, -1) x (0, 1, 0)
ref_plane "to_Bolt_1_386_XY" through (25.3012, 0, 300) normal (0, 1, 0) x (1, 0, 0)
ref_plane "to_Bolt_1_386_YZ" through (25.3012, 0, 300) normal (1, 0, 0) x (0, 0, -1)
ref_plane "to_Bolt_1_386_ZX" through (25.3012, 0, 300) normal (0, 0, -1) x (0, 1, 0)
ref_plane "to_Bolt_1_387_XY" through (27.7108, 0, 300) normal (0, 1, 0) x (1, 0, 0)
ref_plane "to_Bolt_1_387_YZ" through (27.7108, 0, 300) normal (1, 0, 0) x (0, 0, -1)
ref_plane "to_Bolt_1_387_ZX" through (27.7108, 0, 300) normal (0, 0, -1) x (0, 1, 0)
ref_plane "to_Bolt_1_388_XY" through (30.1205, 0, 300) normal (0, 1, 0) x (1, 0, 0)
ref_plane "to_Bolt_1_388_YZ" through (30.1205, 0, 300) normal (1, 0, 0) x (0, 0, -1)
ref_plane "to_Bolt_1_388_ZX" through (30.1205, 0, 300) normal (0, 0, -1) x (0, 1, 0)
ref_plane "to_Bolt_1_389_XY" through (32.5301, 0, 300) normal (0, 1, 0) x (1, 0, 0)
ref_plane "to_Bolt_1_389_YZ" through (32.5301, 0, 300) normal (1, 0, 0) x (0, 0, -1)
ref_plane "to_Bolt_1_389_ZX" through (32.5301, 0, 300) normal (0, 0, -1) x (0, 1, 0)
ref_plane "to_Bolt_1_39_XY" through (-208.4337, 0, -300) normal (0, 1, 0) x (1, 0, 0)
ref_plane "to_Bolt_1_39_YZ" through (-208.4337, 0, -300) normal (1, 0, 0) x (0, 0, -1)
ref_plane "to_Bolt_1_39_ZX" through (-208.4337, 0, -300) normal (0, 0, -1) x (0, 1, 0)
ref_plane "to_Bolt_1_390_XY" through (34.9398, 0, 300) normal (0, 1, 0) x (1, 0, 0)
ref_plane "to_Bolt_1_390_YZ" through (34.9398, 0, 300) normal (1, 0, 0) x (0, 0, -1)
ref_plane "to_Bolt_1_390_ZX" through (34.9398, 0, 300) normal (0, 0, -1) x (0, 1, 0)
ref_plane "to_Bolt_1_391_XY" through (37.3494, 0, 300) normal (0, 1, 0) x (1, 0, 0)
ref_plane "to_Bolt_1_391_YZ" through (37.3494, 0, 300) normal (1, 0, 0) x (0, 0, -1)
ref_plane "to_Bolt_1_391_ZX" through (37.3494, 0, 300) normal (0, 0, -1) x (0, 1, 0)
ref_plane "to_Bolt_1_392_XY" through (39.759, 0, 300) normal (0, 1, 0) x (1, 0, 0)
ref_plane "to_Bolt_1_392_YZ" through (39.759, 0, 300) normal (1, 0, 0) x (0, 0, -1)
ref_plane "to_Bolt_1_392_ZX" through (39.759, 0, 300) normal (0, 0, -1) x (0, 1, 0)
ref_plane "to_Bolt_1_393_XY" through (42.1687, 0, 300) normal (0, 1, 0) x (1, 0, 0)
ref_plane "to_Bolt_1_393_YZ" through (42.1687, 0, 300) normal (1, 0, 0) x (0, 0, -1)
ref_plane "to_Bolt_1_393_ZX" through (42.1687, 0, 300) normal (0, 0, -1) x (0, 1, 0)
ref_plane "to_Bolt_1_394_XY" through (44.5783, 0, 300) normal (0, 1, 0) x (1, 0, 0)
ref_plane "to_Bolt_1_394_YZ" through (44.5783, 0, 300) normal (1, 0, 0) x (0, 0, -1)
ref_plane "to_Bolt_1_394_ZX" through (44.5783, 0, 300) normal (0, 0, -1) x (0, 1, 0)
ref_plane "to_Bolt_1_395_XY" through (46.988, 0, 300) normal (0, 1, 0) x (1, 0, 0)
ref_plane "to_Bolt_1_395_YZ" through (46.988, 0, 300) normal (1, 0, 0) x (0, 0, -1)
ref_plane "to_Bolt_1_395_ZX" through (46.988, 0, 300) normal (0, 0, -1) x (0, 1, 0)
ref_plane "to_Bolt_1_396_XY" through (49.3976, 0, 300) normal (0, 1, 0) x (1, 0, 0)
ref_plane "to_Bolt_1_396_YZ" through (49.3976, 0, 300) normal (1, 0, 0) x (0, 0, -1)
ref_plane "to_Bolt_1_396_ZX" through (49.3976, 0, 300) normal (0, 0, -1) x (0, 1, 0)
ref_plane "to_Bolt_1_397_XY" through (51.8072, 0, 300) normal (0, 1, 0) x (1, 0, 0)
ref_plane "to_Bolt_1_397_YZ" through (51.8072, 0, 300) normal (1, 0, 0) x (0, 0, -1)
ref_plane "to_Bolt_1_397_ZX" through (51.8072, 0, 300) normal (0, 0, -1) x (0, 1, 0)
ref_plane "to_Bolt_1_398_XY" through (54.2169, 0, 300) normal (0, 1, 0) x (1, 0, 0)
ref_plane "to_Bolt_1_398_YZ" through (54.2169, 0, 300) normal (1, 0, 0) x (0, 0, -1)
ref_plane "to_Bolt_1_398_ZX" through (54.2169, 0, 300) normal (0, 0, -1) x (0, 1, 0)
ref_plane "to_Bolt_1_399_XY" through (56.6265, 0, 300) normal (0, 1, 0) x (1, 0, 0)
ref_plane "to_Bolt_1_399_YZ" through (56.6265, 0, 300) normal (1, 0, 0) x (0, 0, -1)
ref_plane "to_Bolt_1_399_ZX" through (56.6265, 0, 300) normal (0, 0, -1) x (0, 1, 0)
ref_plane "to_Bolt_1_4_XY" through (-292.7711, 0, -300) normal (0, 1, 0) x (1, 0, 0)
ref_plane "to_Bolt_1_4_YZ" through (-292.7711, 0, -300) normal (1, 0, 0) x (0, 0, -1)
ref_plane "to_Bolt_1_4_ZX" through (-292.7711, 0, -300) normal (0, 0, -1) x (0, 1, 0)
ref_plane "to_Bolt_1_40_XY" through (-206.0241, 0, -300) normal (0, 1, 0) x (1, 0, 0)
ref_plane "to_Bolt_1_40_YZ" through (-206.0241, 0, -300) normal (1, 0, 0) x (0, 0, -1)
ref_plane "to_Bolt_1_40_ZX" through (-206.0241, 0, -300) normal (0, 0, -1) x (0, 1, 0)
ref_plane "to_Bolt_1_400_XY" through (59.0361, 0, 300) normal (0, 1, 0) x (1, 0, 0)
ref_plane "to_Bolt_1_400_YZ" through (59.0361, 0, 300) normal (1, 0, 0) x (0, 0, -1)
ref_plane "to_Bolt_1_400_ZX" through (59.0361, 0, 300) normal (0, 0, -1) x (0, 1, 0)
ref_plane "to_Bolt_1_401_XY" through (61.4458, 0, 300) normal (0, 1, 0) x (1, 0, 0)
ref_plane "to_Bolt_1_401_YZ" through (61.4458, 0, 300) normal (1, 0, 0) x (0, 0, -1)
ref_plane "to_Bolt_1_401_ZX" through (61.4458, 0, 300) normal (0, 0, -1) x (0, 1, 0)
ref_plane "to_Bolt_1_402_XY" through (63.8554, 0, 300) normal (0, 1, 0) x (1, 0, 0)
ref_plane "to_Bolt_1_402_YZ" through (63.8554, 0, 300) normal (1, 0, 0) x (0, 0, -1)
ref_plane "to_Bolt_1_402_ZX" through (63.8554, 0, 300) normal (0, 0, -1) x (0, 1, 0)
ref_plane "to_Bolt_1_403_XY" through (66.2651, 0, 300) normal (0, 1, 0) x (1, 0, 0)
ref_plane "to_Bolt_1_403_YZ" through (66.2651, 0, 300) normal (1, 0, 0) x (0, 0, -1)
ref_plane "to_Bolt_1_403_ZX" through (66.2651, 0, 300) normal (0, 0, -1) x (0, 1, 0)
ref_plane "to_Bolt_1_404_XY" through (68.6747, 0, 300) normal (0, 1, 0) x (1, 0, 0)
ref_plane "to_Bolt_1_404_YZ" through (68.6747, 0, 300) normal (1, 0, 0) x (0, 0, -1)
ref_plane "to_Bolt_1_404_ZX" through (68.6747, 0, 300) normal (0, 0, -1) x (0, 1, 0)
ref_plane "to_Bolt_1_405_XY" through (71.0843, 0, 300) normal (0, 1, 0) x (1, 0, 0)
ref_plane "to_Bolt_1_405_YZ" through (71.0843, 0, 300) normal (1, 0, 0) x (0, 0, -1)
ref_plane "to_Bolt_1_405_ZX" through (71.0843, 0, 300) normal (0, 0, -1) x (0, 1, 0)
ref_plane "to_Bolt_1_406_XY" through (73.494, 0, 300) normal (0, 1, 0) x (1, 0, 0)
ref_plane "to_Bolt_1_406_YZ" through (73.494, 0, 300) normal (1, 0, 0) x (0, 0, -1)
ref_plane "to_Bolt_1_406_ZX" through (73.494, 0, 300) normal (0, 0, -1) x (0, 1, 0)
ref_plane "to_Bolt_1_407_XY" through (75.9036, 0, 300) normal (0, 1, 0) x (1, 0, 0)
ref_plane "to_Bolt_1_407_YZ" through (75.9036, 0, 300) normal (1, 0, 0) x (0, 0, -1)
ref_plane "to_Bolt_1_407_ZX" through (75.9036, 0, 300) normal (0, 0, -1) x (0, 1, 0)
ref_plane "to_Bolt_1_408_XY" through (78.3133, 0, 300) normal (0, 1, 0) x (1, 0, 0)
ref_plane "to_Bolt_1_408_YZ" through (78.3133, 0, 300) normal (1, 0, 0) x (0, 0, -1)
ref_plane "to_Bolt_1_408_ZX" through (78.3133, 0, 300) normal (0, 0, -1) x (0, 1, 0)
ref_plane "to_Bolt_1_409_XY" through (80.7229, 0, 300) normal (0, 1, 0) x (1, 0, 0)
ref_plane "to_Bolt_1_409_YZ" through (80.7229, 0, 300) normal (1, 0, 0) x (0, 0, -1)
ref_plane "to_Bolt_1_409_ZX" through (80.7229, 0, 300) normal (0, 0, -1) x (0, 1, 0)
ref_plane "to_Bolt_1_41_XY" through (-203.6145, 0, -300) normal (0, 1, 0) x (1, 0, 0)
ref_plane "to_Bolt_1_41_YZ" through (-203.6145, 0, -300) normal (1, 0, 0) x (0, 0, -1)
ref_plane "to_Bolt_1_41_ZX" through (-203.6145, 0, -300) normal (0, 0, -1) x (0, 1, 0)
ref_plane "to_Bolt_1_410_XY" through (83.1325, 0, 300) normal (0, 1, 0) x (1, 0, 0)
ref_plane "to_Bolt_1_410_YZ" through (83.1325, 0, 300) normal (1, 0, 0) x (0, 0, -1)
ref_plane "to_Bolt_1_410_ZX" through (83.1325, 0, 300) normal (0, 0, -1) x (0, 1, 0)
ref_plane "to_Bolt_1_411_XY" through (85.5422, 0, 300) normal (0, 1, 0) x (1, 0, 0)
ref_plane "to_Bolt_1_411_YZ" through (85.5422, 0, 300) normal (1, 0, 0) x (0, 0, -1)
ref_plane "to_Bolt_1_411_ZX" through (85.5422, 0, 300) normal (0, 0, -1) x (0, 1, 0)
ref_plane "to_Bolt_1_412_XY" through (87.9518, 0, 300) normal (0, 1, 0) x (1, 0, 0)
ref_plane "to_Bolt_1_412_YZ" through (87.9518, 0, 300) normal (1, 0, 0) x (0, 0, -1)
ref_plane "to_Bolt_1_412_ZX" through (87.9518, 0, 300) normal (0, 0, -1) x (0, 1, 0)
ref_plane "to_Bolt_1_413_XY" through (90.3614, 0, 300) normal (0, 1, 0) x (1, 0, 0)
ref_plane "to_Bolt_1_413_YZ" through (90.3614, 0, 300) normal (1, 0, 0) x (0, 0, -1)
ref_plane "to_Bolt_1_413_ZX" through (90.3614, 0, 300) normal (0, 0, -1) x (0, 1, 0)
ref_plane "to_Bolt_1_414_XY" through (92.7711, 0, 300) normal (0, 1, 0) x (1, 0, 0)
ref_plane "to_Bolt_1_414_YZ" through (92.7711, 0, 300) normal (1, 0, 0) x (0, 0, -1)
ref_plane "to_Bolt_1_414_ZX" through (92.7711, 0, 300) normal (0, 0, -1) x (0, 1, 0)
ref_plane "to_Bolt_1_415_XY" through (95.1807, 0, 300) normal (0, 1, 0) x (1, 0, 0)
ref_plane "to_Bolt_1_415_YZ" through (95.1807, 0, 300) normal (1, 0, 0) x (0, 0, -1)
ref_plane "to_Bolt_1_415_ZX" through (95.1807, 0, 300) normal (0, 0, -1) x (0, 1, 0)
ref_plane "to_Bolt_1_416_XY" through (97.5904, 0, 300) normal (0, 1, 0) x (1, 0, 0)
ref_plane "to_Bolt_1_416_YZ" through (97.5904, 0, 300) normal (1, 0, 0) x (0, 0, -1)
ref_plane "to_Bolt_1_416_ZX" through (97.5904, 0, 300) normal (0, 0, -1) x (0, 1, 0)
ref_plane "to_Bolt_1_417_XY" through (100, 0, 300) normal (0, 1, 0) x (1, 0, 0)
ref_plane "to_Bolt_1_417_YZ" through (100, 0, 300) normal (1, 0, 0) x (0, 0, -1)
ref_plane "to_Bolt_1_417_ZX" through (100, 0, 300) normal (0, 0, -1) x (0, 1, 0)
ref_plane "to_Bolt_1_418_XY" through (102.4096, 0, 300) normal (0, 1, 0) x (1, 0, 0)
ref_plane "to_Bolt_1_418_YZ" through (102.4096, 0, 300) normal (1, 0, 0) x (0, 0, -1)
ref_plane "to_Bolt_1_418_ZX" through (102.4096, 0, 300) normal (0, 0, -1) x (0, 1, 0)
ref_plane "to_Bolt_1_419_XY" through (104.8193, 0, 300) normal (0, 1, 0) x (1, 0, 0)
ref_plane "to_Bolt_1_419_YZ" through (104.8193, 0, 300) normal (1, 0, 0) x (0, 0, -1)
ref_plane "to_Bolt_1_419_ZX" through (104.8193, 0, 300) normal (0, 0, -1) x (0, 1, 0)
ref_plane "to_Bolt_1_42_XY" through (-201.2048, 0, -300) normal (0, 1, 0) x (1, 0, 0)
ref_plane "to_Bolt_1_42_YZ" through (-201.2048, 0, -300) normal (1, 0, 0) x (0, 0, -1)
ref_plane "to_Bolt_1_42_ZX" through (-201.2048, 0, -300) normal (0, 0, -1) x (0, 1, 0)
ref_plane "to_Bolt_1_420_XY" through (107.2289, 0, 300) normal (0, 1, 0) x (1, 0, 0)
ref_plane "to_Bolt_1_420_YZ" through (107.2289, 0, 300) normal (1, 0, 0) x (0, 0, -1)
ref_plane "to_Bolt_1_420_ZX" through (107.2289, 0, 300) normal (0, 0, -1) x (0, 1, 0)
ref_plane "to_Bolt_1_421_XY" through (109.6386, 0, 300) normal (0, 1, 0) x (1, 0, 0)
ref_plane "to_Bolt_1_421_YZ" through (109.6386, 0, 300) normal (1, 0, 0) x (0, 0, -1)
ref_plane "to_Bolt_1_421_ZX" through (109.6386, 0, 300) normal (0, 0, -1) x (0, 1, 0)
ref_plane "to_Bolt_1_422_XY" through (112.0482, 0, 300) normal (0, 1, 0) x (1, 0, 0)
ref_plane "to_Bolt_1_422_YZ" through (112.0482, 0, 300) normal (1, 0, 0) x (0, 0, -1)
ref_plane "to_Bolt_1_422_ZX" through (112.0482, 0, 300) normal (0, 0, -1) x (0, 1, 0)
ref_plane "to_Bolt_1_423_XY" through (114.4578, 0, 300) normal (0, 1, 0) x (1, 0, 0)
ref_plane "to_Bolt_1_423_YZ" through (114.4578, 0, 300) normal (1, 0, 0) x (0, 0, -1)
ref_plane "to_Bolt_1_423_ZX" through (114.4578, 0, 300) normal (0, 0, -1) x (0, 1, 0)
ref_plane "to_Bolt_1_424_XY" through (116.8675, 0, 300) normal (0, 1, 0) x (1, 0, 0)
ref_plane "to_Bolt_1_424_YZ" through (116.8675, 0, 300) normal (1, 0, 0) x (0, 0, -1)
ref_plane "to_Bolt_1_424_ZX" through (116.8675, 0, 300) normal (0, 0, -1) x (0, 1, 0)
ref_plane "to_Bolt_1_425_XY" through (119.2771, 0, 300) normal (0, 1, 0) x (1, 0, 0)
ref_plane "to_Bolt_1_425_YZ" through (119.2771, 0, 300) normal (1, 0, 0) x (0, 0, -1)
ref_plane "to_Bolt_1_425_ZX" through (119.2771, 0, 300) normal (0, 0, -1) x (0, 1, 0)
ref_plane "to_Bolt_1_426_XY" through (121.6867, 0, 300) normal (0, 1, 0) x (1, 0, 0)
ref_plane "to_Bolt_1_426_YZ" through (121.6867, 0, 300) normal (1, 0, 0) x (0, 0, -1)
ref_plane "to_Bolt_1_426_ZX" through (121.6867, 0, 300) normal (0, 0, -1) x (0, 1, 0)
ref_plane "to_Bolt_1_427_XY" through (124.0964, 0, 300) normal (0, 1, 0) x (1, 0, 0)
ref_plane "to_Bolt_1_427_YZ" through (124.0964, 0, 300) normal (1, 0, 0) x (0, 0, -1)
ref_plane "to_Bolt_1_427_ZX" through (124.0964, 0, 300) normal (0, 0, -1) x (0, 1, 0)
ref_plane "to_Bolt_1_428_XY" through (126.506, 0, 300) normal (0, 1, 0) x (1, 0, 0)
ref_plane "to_Bolt_1_428_YZ" through (126.506, 0, 300) normal (1, 0, 0) x (0, 0, -1)
ref_plane "to_Bolt_1_428_ZX" through (126.506, 0, 300) normal (0, 0, -1) x (0, 1, 0)
ref_plane "to_Bolt_1_429_XY" through (128.9157, 0, 300) normal (0, 1, 0) x (1, 0, 0)
ref_plane "to_Bolt_1_429_YZ" through (128.9157, 0, 300) normal (1, 0, 0) x (0, 0, -1)
ref_plane "to_Bolt_1_429_ZX" through (128.9157, 0, 300) normal (0, 0, -1) x (0, 1, 0)
ref_plane "to_Bolt_1_43_XY" through (-198.7952, 0, -300) normal (0, 1, 0) x (1, 0, 0)
ref_plane "to_Bolt_1_43_YZ" through (-198.7952, 0, -300) normal (1, 0, 0) x (0, 0, -1)
ref_plane "to_Bolt_1_43_ZX" through (-198.7952, 0, -300) normal (0, 0, -1) x (0, 1, 0)
ref_plane "to_Bolt_1_430_XY" through (131.3253, 0, 300) normal (0, 1, 0) x (1, 0, 0)
ref_plane "to_Bolt_1_430_YZ" through (131.3253, 0, 300) normal (1, 0, 0) x (0, 0, -1)
ref_plane "to_Bolt_1_430_ZX" through (131.3253, 0, 300) normal (0, 0, -1) x (0, 1, 0)
ref_plane "to_Bolt_1_431_XY" through (133.7349, 0, 300) normal (0, 1, 0) x (1, 0, 0)
ref_plane "to_Bolt_1_431_YZ" through (133.7349, 0, 300) normal (1, 0, 0) x (0, 0, -1)
ref_plane "to_Bolt_1_431_ZX" through (133.7349, 0, 300) normal (0, 0, -1) x (0, 1, 0)
ref_plane "to_Bolt_1_432_XY" through (136.1446, 0, 300) normal (0, 1, 0) x (1, 0, 0)
ref_plane "to_Bolt_1_432_YZ" through (136.1446, 0, 300) normal (1, 0, 0) x (0, 0, -1)
ref_plane "to_Bolt_1_432_ZX" through (136.1446, 0, 300) normal (0, 0, -1) x (0, 1, 0)
ref_plane "to_Bolt_1_433_XY" through (138.5542, 0, 300) normal (0, 1, 0) x (1, 0, 0)
ref_plane "to_Bolt_1_433_YZ" through (138.5542, 0, 300) normal (1, 0, 0) x (0, 0, -1)
ref_plane "to_Bolt_1_433_ZX" through (138.5542, 0, 300) normal (0, 0, -1) x (0, 1, 0)
ref_plane "to_Bolt_1_434_XY" through (140.9639, 0, 300) normal (0, 1, 0) x (1, 0, 0)